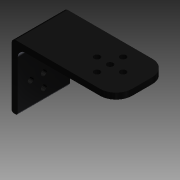
# Autodesk Inventor part: L_micro_sergei_dines
Saved by Autodesk Inventor 2014 SP2 (Build 180246200, 246)
## iProperties
Created: 2014-12-14
Part Number: L_micro_sergei_dines
Material: Generic
Document SubType Name: Modeling
Designer: Sergei
Density: 1 g/cm^3
Appearance: Glossy - Black
Author: Sergei
Autodesk Inventor part; units mm, degrees
ref_plane "YZ Plane" through (0, 0, 0) normal (1, 0, 0) x (0, 1, 0)
ref_plane "XZ Plane" through (0, 0, 0) normal (0, 1, 0) x (-1, 0, 0)
ref_plane "XY Plane" through (0, 0, 0) normal (0, 0, 1) x (1, 0, 0)
sketch "Sketch1" plane through (0, 0, 0) normal (0, 0, 1) x (1, 0, 0)
  line L0 (0, 0) -> (-49, 0)
  line L1 (-49, 0) -> (-49, 18)
  line L2 (-49, 18) -> (0, 18) construction
  line L3 (-49, 18) -> (-52, 18)
  line L4 (-52, 18) -> (-52, -3)
  line L5 (-52, -3) -> (0, -3)
  line L6 (0, -3) -> (0, 0)
  dimension "d0" = 18
  dimension "d1" = 3
  dimension "d2" = 3
  dimension "d3" = 52
  constraints: 14 end point, 5 perpendicular, 1 coincident, 1 horizontal
  measures "d0" distance between parallel lines of L2 L0
  measures "d1" distance between parallel lines of L4 L1
  measures "d2" distance between parallel lines of L5 L0
  measures "d3" distance between parallel lines of L6 L4
extrude "Extrusion1" add sketch "Sketch1" along normal blind 10
mirror "Mirror1" about plane through (-32.0411, 1.4589, 0) normal (0, 0, -1) of "Extrusion1"
mirror "Mirror2" about plane through (-49, 18, 0) normal (0, 1, 0) of "Extrusion1", "Mirror1"
sketch "Sketch4" plane through (0, -3, -10) normal (0, 0, -1) x (-1, 0, 0)
  line L0 (0, 3) -> (49, 3) projected
  line L1 (0, 0) -> (0, 3) projected
  line L2 (52, 0) -> (0, 0) projected
  line L3 (52, 42) -> (52, 0) projected
  line L4 (52, 42) -> (0, 42) projected
  line L5 (0, 42) -> (0, 39) projected
  line L6 (0, 39) -> (49, 39) projected
  line L7 (49, 39) -> (49, 3) projected
  line L8 (0, 3) -> (49, 3) projected
  line L9 (0, 0) -> (0, 3) projected
  line L10 (52, 0) -> (0, 0) projected
  line L11 (52, 42) -> (52, 0) projected
  line L12 (52, 42) -> (0, 42) projected
  line L13 (0, 42) -> (0, 39) projected
  line L14 (0, 39) -> (49, 39) projected
  line L15 (49, 39) -> (49, 3) projected
extrude "Extrusion4" add sketch "Sketch4" along normal blind 5
mirror "Mirror3" about plane through (0, 0, 0) normal (0, 0, 1) of "Extrusion4"
sketch "Sketch11" plane through (-52, -3, -15) normal (0, -1, 0) x (1, 0, 0)
  line L0 (52, 0) -> (52, 30) projected
  line L1 (52, 30) -> (0, 30) projected
  line L2 (0, 0) -> (0, 30) projected
  line L3 (52, 0) -> (0, 0) projected
  line L4 (52, 0) -> (52, 30) projected
  line L5 (52, 30) -> (0, 30) projected
  line L6 (0, 0) -> (0, 30) projected
  line L7 (52, 0) -> (0, 0) projected
  point P0 (52, 15)
extrude "Extrusion11" cut sketch "Sketch11" against normal blind 10
sketch "Sketch13" plane through (0, 36, -15) normal (1, 0, 0) x (0, 0, -1)
  line L0 (-30, 3) -> (-28, 3)
  line L1 (-28, 3) -> (-28, -29)
  line L2 (-28, -29) -> (-30, -29)
  line L3 (-30, -29) -> (-30, 3)
  line L4 (-30, -29) -> (0, -29) projected
  point P0 (-15, -36)
  dimension "d65" = 2
  constraints: 8 end point, 2 parallel, 1 collinear, 1 horizontal, 1 perpendicular
  measures "d65" distance of L1.end L2.end
extrude "Extrusion13" cut sketch "Sketch13" against normal up to next
mirror "Mirror4" about plane through (0, 0, 0) normal (0, 0, 1) of "Extrusion13"
sketch "Sketch14" plane through (-52, 7, 13) normal (-1, 0, 0) x (0, 0, 1)
  line L0 (-26, 32) -> (-26, 0) projected
  line L1 (-26, 0) -> (0, 0) projected
  line L2 (0, 32) -> (-26, 32) projected
  circle A0 centre (-13, 12) radius 6.5 construction
  line L3 (-13, 12) -> (-26, 12) construction
  line L4 (-13, 12) -> (-13, 32) construction
  circle A1 centre (-13, 12) radius 1.5
  circle A2 centre (-13, 18.5) radius 1.5
  point P0 (-13, -7)
  point P1 (-13, 0)
  dimension "d68" = 13
  dimension "d69" = 20
  dimension "d71" = 3
  dimension "d72" = 3
  constraints: 4 end point, 2 centre point, 2 midpoint, 2 point on line, 2 vertical alignment, 1 coincident, 1 parallel, 1 perpendicular, 2 other
  measures "d69" distance between parallel lines of L2 L3
  measures "d71" diameter of A2
  measures "d72" diameter of A1
extrude "Extrusion14" cut sketch "Sketch14" against normal up to next
pattern_circular "Circular Pattern6" count 4 over 360 about axis through (-52, 19, 0) along (1, 0, 0) of "Extrusion14"
sketch "Sketch15" plane through (-49, 36, 13) normal (0, -1, 0) x (1, 0, 0)
  line L0 (49, -26) -> (49, 0) projected
  line L1 (49, 0) -> (0, 0) projected
  circle A0 centre (33, -13) radius 6.5 construction
  line L2 (33, -13) -> (33, 0) construction
  circle A1 centre (33, -6.5) radius 1.5
  circle A2 centre (33, -13) radius 1.5
  point P0 (49, -13)
  point P1 (49, -13)
  dimension "d78" = 13
  dimension "d79" = 16
  dimension "d80" = 3
  dimension "d81" = 3
  constraints: 3 centre point, 2 coincident, 2 end point, 2 midpoint, 1 horizontal alignment, 1 parallel, 1 perpendicular, 1 point on line
  measures "d78" diameter of A0
  measures "d79" distance between parallel lines of L0 L2
  measures "d80" diameter of A1
  measures "d81" diameter of A2
extrude "Extrusion15" cut sketch "Sketch15" against normal up to next
pattern_circular "Circular Pattern7" count 4 over 360 about axis through (-16, 36, 0) along (0, 1, 0) of "Extrusion15"
fillet "Fillet1" radius 8 2 edges at (0, 37.5, -13) (0, 37.5, 13)
sketch "Sketch18" plane through (-52, 39, 13) normal (0, 1, 0) x (1, 0, 0)
  arc A0 (44, 0) -> (52, 8) centre (44, 8) ccw projected
  line L0 (52, 8) -> (52, 18) projected
  arc A1 (52, 18) -> (44, 26) centre (44, 18) ccw projected
  line L1 (44, 26) -> (0, 26) projected
  line L2 (0, 0) -> (0, 26) projected
  line L3 (0, 0) -> (44, 0) projected
  circle A2 centre (36, 13) radius 1.5 projected
  circle A3 centre (36, 6.5) radius 1.5 projected
  circle A4 centre (29.5, 13) radius 1.5 projected
  circle A5 centre (42.5, 13) radius 1.5 projected
  circle A6 centre (36, 19.5) radius 1.5 projected
  point P0 (52, 13)
  dimension "d93" = 26
  measures "d93" distance of L2.start L1.end
fillet "Fillet2" radius 4 1 edges at (-49, 36, 0)
fillet "Fillet3" radius 2 1 edges at (-52, 39, 0)
fillet "Fillet4" radius 1 2 edges at (-49, 7, 0) (-52, 7, 0)
equation "\"d72\" = d71"
body "Solid1"
